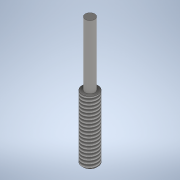
# Autodesk Inventor part: burner rodx3 part 1
Saved by Autodesk Inventor 2020 (Build 240168000, 168)
## iProperties
Created: 2019-06-12
Part Number: burner rodx3 part 1
Material: Stainless Steel
Document SubType Name: Modeling
Designer: ColinP
Density: 8 g/cm^3
Appearance: Semi-Polished
Author: ColinP
Autodesk Inventor part; units mm, degrees
ref_plane "YZ Plane" through (0, 0, 0) normal (1, 0, 0) x (0, 1, 0)
ref_plane "XZ Plane" through (0, 0, 0) normal (0, 1, 0) x (-1, 0, 0)
ref_plane "XY Plane" through (0, 0, 0) normal (0, 0, 1) x (1, 0, 0)
sketch "Sketch1" plane through (0, 0, 0) normal (0, 1, 0) x (-1, 0, 0)
  circle A0 centre (0, 0) radius 1.5875
  dimension "d0" = 3.175
  constraints: 1 centre point, 1 coincident
  measures "d0" diameter of A0
extrude "Extrusion1" add sketch "Sketch1" along normal blind 12.7
thread "Thread1" size "5-40 UNC" class "2A" standard "ANSI Unified Screw Threads" length 12.7
chamfer "Chamfer1" distance 0.254 angle 45 1 edges at (1.5875, 0, 0)
sketch "Sketch3" plane through (0, 12.7, 0) normal (0, 1, 0) x (1, 0, 0)
  circle A0 centre (0, 0) radius 0.9525
  dimension "d11" = 1.905
  constraints: 1 centre point, 1 coincident
  measures "d11" diameter of A0
extrude "Extrusion3" add sketch "Sketch3" along normal blind 12.7
body "Solid1"
